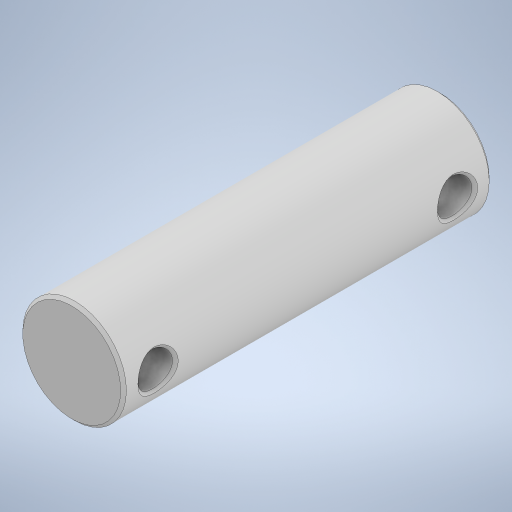
# Autodesk Inventor part: 05-16-2023 Perno
Saved by Autodesk Inventor 2023 (Build 270158000, 158)
## iProperties
Created: 2023-05-16
Part Number: 05-16-2023 Perno
Material: Generico
Document SubType Name: Modeling
Designer: Admin
Density: 1 g/cm^3
Appearance: Default
Author: Admin
Autodesk Inventor part; units mm, degrees
ref_plane "YZ Plane" through (0, 0, 0) normal (1, 0, 0) x (0, 1, 0)
ref_plane "XZ Plane" through (0, 0, 0) normal (0, 1, 0) x (-1, 0, 0)
ref_plane "XY Plane" through (0, 0, 0) normal (0, 0, 1) x (1, 0, 0)
sketch "Schizzo1" plane through (0, 0, 0) normal (0, 0, 1) x (1, 0, 0)
  circle A0 centre (0, 0) radius 9
  dimension "d2" = 18
  constraints: 1 centre point, 1 coincident
  measures "d2" diameter of A0
extrude "Estrusione1" add sketch "Schizzo1" along normal mid plane 64
sketch "Schizzo2" plane through (0, 0, 0) normal (1, 0, 0) x (0, 1, 0)
  line L0 (0, 0) -> (0, -36.2228) construction
  line L1 (0, 0) -> (14.2779, 0) construction
  point P0 (0, -26)
  point P1 (0, 26)
  dimension "d3" = 52
  constraints: 4 end point, 1 horizontal, 1 point on line, 1 symmetric about line, 1 vertical
  measures "d3" distance of point (0, -26) point (0, 26)
hole "Foro1" at (0, 0, -26) at (0, 0, 26) direction (-1, 0, 0) diameter 6 end through all both
chamfer "Smusso1" distance 0.5 angle 45 8 edges at (-9, 0, 32) (-9, 0, -32) (8.4853, -3, 25.9929) (8.4853, 3, 26.0071) (8.4853, 3, -25.9929) (8.4853, -3, -26.0071) (-9, 0.0262, -23.0001) (-9, 0.0262, 28.9999)
